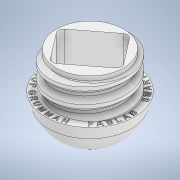
# Autodesk Inventor part: SmartEgg Shell
Saved by Autodesk Inventor 2020 (Build 240168000, 168)
## iProperties
Created: 2019-11-26
Part Number: SmartEgg Shell
Material: Generic
Document SubType Name: Modeling
Designer: Andrew
Density: 1 g/cm^3
Appearance: White
d0: 1.000 ul
d17: 1.000 ul
d18: 25.000 mm
d19: 50.000 mm
d20: 1.000 mm
d21: 17.000 mm
d22: 5.000 mm
d23: 2.000 mm
d24: 12.500 mm
d25: 0.250 mm
d26: 20.000 mm
d27: 3.000 mm
d28: 1.500 mm
d30: 1.000 mm
d32: 0.500 mm
d33: 0.500 mm
d35: 45.00 deg
d36: 0.250 mm
d37: 2.000 mm
d38: 2.000 mm
d41: 8.708 mm
d43: 3.000 ul
d44: 0.00 deg
d50: 8.708 mm
d52: 1.000 ul
d53: 0.00 deg
d61: 2.500 mm
d29: 70.533 mm
d39: 7.000 mm
Thread_Pitch: 4.354 mm
BATT_Width: 24.750 mm
PCB_Width: 22.950 mm
Author: Andrew
Autodesk Inventor part; units mm, degrees
ref_plane "YZ Plane" through (0, 0, 0) normal (1, 0, 0) x (0, 1, 0)
ref_plane "XZ Plane" through (0, 0, 0) normal (0, 1, 0) x (-1, 0, 0)
ref_plane "XY Plane" through (0, 0, 0) normal (0, 0, 1) x (1, 0, 0)
derived "SmartEgg Housing Main.ipt"
sketch "Sketch3" plane through (0, 0, 0) normal (0, 0, 1) x (1, 0, 0)
  line L0 (25.5, 9.7) -> (25.5, -9.55)
  line L1 (26.5, 11.95) -> (26.5, -11.8)
  line L2 (-26.5, -11.8) -> (-26.5, 11.95)
  line L3 (-7.3114, 6.9165) -> (-15.25, -6.8335)
  line L4 (-15.5, -6.7665) -> (-7.5614, 6.9835)
  line L5 (-26.5, 11.95) -> (-7.5614, 11.95)
  line L6 (-7.3114, 11.95) -> (26.5, 11.95)
  line L7 (-25.5, 9.7) -> (7.4386, 9.7)
  line L8 (7.6886, 9.7) -> (25.5, 9.7)
  line L9 (25.5, -9.55) -> (-0.25, -9.55)
  line L10 (-0.5, -9.55) -> (-25.5, -9.55)
  line L11 (26.5, -11.8) -> (-15.25, -11.8)
  line L12 (-15.5, -11.8) -> (-26.5, -11.8)
  line L13 (25.5, 0) -> (25.5, -1.8) construction
  line L14 (-25.5, -1.8) -> (-25.5, 0) construction
  line L15 (-25.5, -3.3) -> (-0.5, -3.3)
  line L16 (-0.5, -3.3) -> (-0.5, -4.3)
  line L17 (-0.5, -4.3) -> (-25.5, -4.3)
  line L18 (-25.5, -9.55) -> (-25.5, -4.3)
  line L19 (-25.5, -3.3) -> (-25.5, 9.7)
  line L20 (-7.4364, 11.95) -> (-7.4364, 6.95) construction
  line L21 (-7.4364, 6.95) -> (-15.375, -6.8) construction
  line L22 (-15.375, -6.8) -> (-15.375, -11.8) construction
  line L23 (-7.5614, 11.95) -> (-7.5614, 10.7)
  line L24 (-7.5614, 10.7) -> (7.4386, 10.7)
  line L25 (7.4386, 10.7) -> (7.4386, 9.7)
  line L26 (7.6886, 9.7) -> (7.6886, 10.95)
  line L27 (7.6886, 10.95) -> (-7.3114, 10.95)
  line L28 (-7.3114, 10.95) -> (-7.3114, 11.95)
  line L29 (-15.5, -11.8) -> (-15.5, -10.55)
  line L30 (-15.5, -10.55) -> (-0.5, -10.55)
  line L31 (-0.5, -10.55) -> (-0.5, -9.55)
  line L32 (-0.25, -9.55) -> (-0.25, -10.8)
  line L33 (-0.25, -10.8) -> (-15.25, -10.8)
  line L34 (-15.25, -10.8) -> (-15.25, -11.8)
  line L35 (-7.5614, 10.7) -> (-7.5614, 6.9835)
  line L36 (-7.3114, 6.9165) -> (-7.3114, 10.95)
  line L37 (-15.5, -10.55) -> (-15.5, -6.7665)
  line L38 (-15.25, -6.8335) -> (-15.25, -10.8)
  line L39 (7.4386, 9.7) -> (7.4386, 6.9835)
  line L40 (7.4386, 6.9835) -> (-0.5, -6.7665)
  line L41 (-0.5, -6.7665) -> (-0.5, -9.55)
  line L42 (-0.25, -9.55) -> (-0.25, -6.8335)
  line L43 (-0.25, -6.8335) -> (7.6886, 6.9165)
  line L44 (7.6886, 6.9165) -> (7.6886, 9.7)
  line L45 (-0.375, -11.8) -> (-0.375, -6.8) construction
  line L46 (-0.375, -6.8) -> (7.5636, 6.95) construction
  line L47 (7.5636, 6.95) -> (7.5636, 11.95) construction
  line L48 (11.5, -9.55) -> (16.5, -9.55)
  line L49 (16.5, -9.55) -> (14, -7.05)
  line L50 (14, -7.05) -> (11.5, -7.05)
  line L51 (11.5, -7.05) -> (11.5, -9.55)
  point P0 (0, 0)
derived "SmartEgg Housing Cap.ipt"
sketch "Housing Largest Area" plane through (0, -10.6204, -14.0095) normal (0, 0.7948428, -0.6068154) x (0, 0.6068154, 0.7948428)
  line L0 (30.7511, 26.5) -> (29.3995, 26.5)
  line L1 (17.6255, 26.5) -> (17.6255, -26.5)
  line L2 (17.6255, -26.5) -> (35.2511, -26.5)
  line L3 (35.2511, -26.5) -> (35.2511, 22)
  line L4 (10.4196, -26.5) -> (24.8315, -26.5) construction
  line L5 (24.8315, 26.5) -> (10.4196, 26.5) construction
  line L6 (12.0637, 20.5) -> (10.4158, 20.5) construction
  line L7 (10.4158, 20.5) -> (10.4158, 24.5) construction
  ellipse E0 centre (8.7678, 24.5) end of major axis (10.4158, 24.5) minor radius 1 (10.4158, 24.5) -> (8.7678, 25.5) ccw construction
  line L8 (8.7678, 25.5) -> (2.3515, 25.5) construction
  line L9 (2.3515, 25.5) -> (2.3515, 16.1435) construction
  line L10 (2.3515, -0.25) -> (1, -0.25) construction
  line L11 (1, -0.25) -> (1, -15.25) construction
  line L12 (1, -15.25) -> (0, -15.25) construction
  line L13 (0, -15.25) -> (0, 26.5) construction
  line L14 (17.0488, 25.5) -> (14.5356, 25.5) construction
  line L15 (14.5356, 25.5) -> (14.5356, 22.4142) construction
  ellipse E1 centre (12.8877, 22.4142) end of major axis (14.5356, 22.4142) minor radius 1 (14.053, 21.7071) -> (14.5356, 22.4142) ccw construction
  line L16 (14.053, 21.7071) -> (12.0637, 20.5) construction
  line L17 (35.2511, 26.5) -> (35.2511, -7.3114) construction
  line L18 (35.2511, -7.3114) -> (34.2511, -7.3114) construction
  line L19 (34.2511, -7.3114) -> (34.2511, 7.6886) construction
  line L20 (34.2511, 7.6886) -> (32.8995, 7.6886) construction
  line L21 (32.8995, 7.6886) -> (32.8995, 25.5) construction
  arc A0 (35.2511, 22) -> (30.7511, 26.5) centre (30.7511, 22) ccw
  arc A1 (32.8995, 22) -> (29.3995, 25.5) centre (29.3995, 22) ccw
  line L22 (32.8995, 22) -> (35.2511, 22)
  line L23 (29.3995, 25.5) -> (29.3995, 26.5)
  line L24 (29.3995, 26.5) -> (17.6255, 26.5)
  line L25 (2.3515, 16.1435) -> (4.5726, 14.7957)
  line L26 (4.5726, 14.7957) -> (4.5726, 11.5)
  line L27 (4.5726, 11.5) -> (2.3515, 11.5)
  line L28 (2.3515, 11.5) -> (2.3515, -0.25)
  line L29 (0, 26.5) -> (17.0488, 26.5)
  line L30 (17.0488, 26.5) -> (17.0488, 25.5)
  line L31 (32.8995, 25.5) -> (21.9926, 25.5)
  line L32 (21.9926, 25.5) -> (21.9926, 26.5)
  line L33 (21.9926, 26.5) -> (35.2511, 26.5)
  point P0 (17.58, 0)
  point P1 (17.6255, 0)
sketch "ESP32 Feather" plane through (0, 0, 0) normal (0, 0, 1) x (1, 0, 0)
  line L0 (-25.5, 0) -> (25.5, 0)
  line L1 (25.5, 0) -> (25.5, -1.8)
  line L2 (25.5, -1.8) -> (-25.5, -1.8)
  line L3 (-25.5, -1.8) -> (-25.5, 0)
  line L4 (0, 0) -> (-25.5, 0)
  line L5 (-25.5, 0) -> (-25.5, 0.75)
  line L6 (-25.5, 0.75) -> (0, 0.75)
  line L7 (0, 0.75) -> (0, 0)
  line L8 (-0.9, 0.75) -> (-18.55, 0.75)
  line L9 (-18.55, 0.75) -> (-18.55, 3.1)
  line L10 (-18.55, 3.1) -> (-0.9, 3.1)
  line L11 (-0.9, 3.1) -> (-0.9, 0.75)
  line L12 (10, 0) -> (18, 0)
  line L13 (18, 0) -> (18, 5.5)
  line L14 (18, 5.5) -> (10, 5.5)
  line L15 (10, 5.5) -> (10, 0)
  line L16 (25.6, 0) -> (19.95, 0)
  line L17 (19.95, 0) -> (19.95, 2.45)
  line L18 (19.95, 2.45) -> (25.6, 2.45)
  line L19 (25.6, 2.45) -> (25.6, 0)
  point P0 (0, 0)
  point P1 (0, 0)
  point P2 (-18.55, 0.75)
  point P3 (18, 0)
  point P4 (19.95, 0)
sketch "Shell Sketch" plane through (0, -10.6204, -14.0095) normal (0, 0.7948428, -0.6068154) x (0, 0.6068154, 0.7948428)
  arc A0 (41.0761, -18.875) -> (29.7061, 33.6321) centre (-5.8251, -1.5465) ccw
  arc A1 (17.6255, -35.2107) -> (30.1255, -31.8614) centre (17.6255, -10.2107) ccw construction
  line L0 (17.6255, -35.2107) -> (17.6255, -31.8614) construction
  line L1 (17.6255, 9) -> (36.7511, 9)
  line L2 (17.6255, 26.5) -> (17.6255, -26.5) construction
  line L3 (35.2511, -26.5) -> (35.9855, -27.1787) construction
  arc A2 (29.7061, 33.6321) -> (17.6255, 38.6714) centre (17.6255, 21.6714) ccw
  line L4 (17.6255, 38.6714) -> (17.6255, 35.8135)
  line L5 (17.6255, 35.8135) -> (22.6255, 35.8135)
  arc A3 (28.2849, 32.225) -> (22.6255, 35.8135) centre (17.6255, 21.6714) ccw
  arc A4 (37.3586, 19.41) -> (28.2849, 32.225) centre (-5.8251, -1.5465) ccw
  arc A5 (35.2511, 22) -> (30.7511, 26.5) centre (30.7511, 22) ccw construction
  line L6 (36.7511, 9) -> (36.7511, -11.8614)
  line L7 (36.7511, -11.8614) -> (43.0994, -11.8614)
  line L8 (39.7511, 9) -> (39.7511, -11.6114)
  line L9 (39.7511, -11.6114) -> (43.1514, -11.6114)
  line L10 (17.6255, -31.8614) -> (30.1255, -31.8614)
  arc A6 (30.1255, -31.8614) -> (41.0761, -18.875) centre (17.6255, -10.2107) ccw
  line L11 (17.6255, -31.8614) -> (17.6255, 9)
  line L12 (35.2511, -26.5) -> (35.2511, 22) construction
  line L13 (20.9175, 10) -> (17.58, 10) construction
  arc A7 (39.7511, 9) -> (37.3586, 19.41) centre (15.9074, 9) ccw
  point P0 (17.58, 0)
  point P1 (39.7511, 13.5139)
  dimension "d18" = 25
  dimension "d19" = 50
  dimension "d20" = 1
  dimension "d21" = 17
  dimension "d22" = 5
  dimension "d23" = 2
  dimension "d24" = 12.5
  dimension "d25" = 0.25
  dimension "d26" = 20
  dimension "d27" = 3
  dimension "d28" = 1.5
  dimension "d29" = 70.5327
  dimension "d30" = 1
  constraints: 22 end point, 19 point on circle, 7 centre point, 7 line through centre, 6 perpendicular, 6 tangent, 4 collinear, 4 vertical, 2 concentric, 2 point on line, 1 coincident, 1 horizontal
  measures "d18" radius of A1
  measures "d19" radius of A0
  measures "d20" distance of L3.start L3.end
  measures "d21" radius of A2
  measures "d22" distance of L4.end L5.end
  measures "d23" radial gap between concentric circles of A0 A4
  measures "d24" distance of L0.end L10.end
  measures "d25" distance between parallel lines of L7 L9
  measures "d26" distance between parallel lines of L10 L7
  measures "d27" distance between parallel lines of L8 L6
  measures "d28" distance between parallel lines of L12 L6
  measures "d29" distance from line of L10 L4.start
  measures "d30" distance between parallel lines of L1 L13
sketch "Thread Sketch" plane through (0, -10.6204, -14.0095) normal (0, 0.7948428, -0.6068154) x (0, 0.6068154, 0.7948428)
  line L0 (36.7511, 9) -> (36.7511, -11.8614) construction
  line L1 (39.7511, 9) -> (39.7511, -11.6114) construction
  line L2 (36.7511, 9) -> (39.2511, 6.5)
  line L3 (39.2511, 6.5) -> (39.2511, 4.5)
  line L4 (39.2511, 4.5) -> (36.7511, 2)
  line L5 (36.7511, 2) -> (36.7511, 9)
  line L6 (39.7511, 4.6464) -> (37.2511, 2.1464)
  line L7 (37.2511, 2.1464) -> (37.2511, 0.1464)
  line L8 (37.2511, 0.1464) -> (39.7511, -2.3536)
  line L9 (39.7511, -2.3536) -> (39.7511, 4.6464)
  line L10 (39.2511, 5.5) -> (36.7511, 5.5) construction
  line L11 (37.2511, 1.1464) -> (39.7511, 1.1464) construction
  point P0 (17.58, 0)
  dimension "d32" = 0.5
  dimension "d33" = 0.5
  dimension "d35" = 45
  dimension "d36" = 0.25
  dimension "d37" = 2
  dimension "d38" = 2
  dimension "d39" = 7
  dimension "Thread_Pitch" = 4.354
  constraints: 20 end point, 4 midpoint, 3 parallel, 2 horizontal, 2 point on line, 2 other
  measures "d32" distance between parallel lines of L1 L3
  measures "d33" distance between parallel lines of L0 L7
  measures "d35" angle of L0 L4
  measures "d36" distance between parallel lines of L6 L4
  measures "d37" distance of L2.end L3.end
  measures "d38" distance of L6.end L7.end
  measures "d39" distance of L4.end L0.start
revolve "Revolution1" add sketch "Shell Sketch" angle 360 about axis through (-31.8614, 0.075, 0) along (1, 0, 0) contours A6 L10 L11 L1 L6 L7 A0
coil "Coil1" sketch "Thread Sketch" operation add axis through (-31.8614, 0.075, 0) along (-1, 0, 0) pitch 8.708 turns 3 hand right separate body contours L2 L3 L4 L5
coil "Coil2" sketch "Thread Sketch" operation add axis through (-31.8614, 0.075, 0) along (1, 0, 0) pitch 8.708 turns 1 hand right bodies 2 contours L2 L3 L4 L5
sketch "Thread Mask" plane through (0, -10.6204, -14.0095) normal (0, 0.7948428, -0.6068154) x (0, 0.6068154, 0.7948428)
  line L0 (39.7511, 6.5) -> (36.7511, 6.5)
  line L1 (36.7511, 6.5) -> (36.7511, -11.8614)
  line L2 (36.7511, -11.8614) -> (39.7511, -11.8614)
  line L3 (39.7511, -11.8614) -> (39.7511, 6.5)
  line L4 (36.7511, 9) -> (36.7511, -11.8614) construction
  line L5 (39.7511, 9) -> (39.7511, -11.6114) construction
  point P0 (17.58, 0)
  dimension "d61" = 2.5
  constraints: 8 end point, 2 parallel, 1 collinear, 1 horizontal, 1 perpendicular
  measures "d61" distance from line of L4.start L0
revolve "Revolution4" cut sketch "Thread Mask" angle 360 about axis through (-31.8614, 0.075, 0) along (1, 0, 0) keep common part bodies 2
combine bodies "Combine1" operation type add bodies to combine 1 2
sketch "Sketch10" plane through (9, 0.075, 0) normal (1, 0, 0) x (0, 0, -1)
  line L0 (-11.875, -12.125) -> (11.875, -12.125)
  line L1 (14.875, -9.125) -> (14.875, 9.125)
  line L2 (11.875, 12.125) -> (-11.875, 12.125)
  line L3 (-14.875, 9.125) -> (-14.875, -9.125)
  line L4 (-14.875, 0) -> (14.875, 0) construction
  arc A0 (-11.875, 12.125) -> (-14.875, 9.125) centre (-11.875, 9.125) ccw
  arc A1 (14.875, 9.125) -> (11.875, 12.125) centre (11.875, 9.125) ccw
  arc A2 (11.875, -12.125) -> (14.875, -9.125) centre (11.875, -9.125) ccw
  arc A3 (-14.875, -9.125) -> (-11.875, -12.125) centre (-11.875, -9.125) ccw
  point P0 (0, -0.075)
  point P1 (14.875, 12.125)
  point P2 (-14.875, 12.125)
  point P3 (0, -11.875)
  point P4 (0, -11.875)
  point P5 (0, -11.875)
  point P6 (0, 11.875)
  point P7 (0, 11.875)
  point P8 (0, 11.875)
  point P9 (0, 0)
  point P10 (0, 0)
  point P11 (0, 0)
  point P12 (0, 0)
  dimension "d64" = 0.25
  dimension "d65" = 29.75
  dimension "d66" = 3
  constraints: 10 end point, 8 point on circle, 8 tangent, 4 centre point, 4 point on line, 3 equal radius, 3 midpoint, 2 parallel, 1 coincident, 1 horizontal, 1 perpendicular
  measures "d64" distance from line of L0 point (0, -11.875)
  measures "d65" distance of point (14.875, 12.125) point (-14.875, 12.125)
  measures "d66" radius of A0
sketch "Sketch11" plane through (0, 0, 0) normal (0, 0, 1) x (1, 0, 0)
  line L0 (9, 19.2005) -> (9, -19.0505) projected
  line L1 (9, 0.075) -> (-26.5, 0.075)
  line L2 (-26.5, -11.8) -> (-26.5, 11.95) construction
  point P0 (0, 0)
  dimension "d67" = 35.5
  constraints: 2 end point, 2 midpoint, 1 horizontal
  measures "d67" distance of L1.start L1.end
extrude "Extrusion1" cut sketch "Sketch10" against normal blind 35.5 bodies 1
sketch "Vent Lookup" plane through (0, -10.6204, -14.0095) normal (0, 0.7948428, -0.6068154) x (0, 0.6068154, 0.7948428)
  arc A0 (41.0761, -18.875) -> (29.7061, 33.6321) centre (-5.8251, -1.5465) ccw projected
  line L0 (40.8046, 16.5) -> (17.6255, 7.5293)
  line L1 (17.6255, 26.5) -> (17.6255, -26.5) construction
  line L2 (20.9175, 10) -> (17.58, 10) construction
  point P0 (17.58, 0)
  dimension "d71" = 6.5
  constraints: 2 end point, 1 line through centre, 1 point on circle, 1 point on line
  measures "d71" distance from line of L2 L0.start
ref_plane "Vent Plane" through (16.5, 14.1404, 18.4237) normal (-0.3609294, -0.5659119, -0.7412649) x (0.8431188, -0.5377274, 0)
sketch "Sketch13" plane through (-11.8614, 0.075, 0) normal (1, 0, 0) x (0, 0, -1)
  circle A0 centre (0, -0.075) radius 24.75 construction
  line L0 (7.0609, -23.8279) -> (6.0494, -20.9526)
  line L1 (6.0494, -20.9526) -> (6.6126, -20.7545)
  line L2 (6.6126, -20.7545) -> (8.4723, -22.2675)
  line L3 (8.4723, -22.2675) -> (7.7938, -20.3389)
  line L4 (7.7938, -20.3389) -> (8.3307, -20.15)
  line L5 (8.3307, -20.15) -> (9.3423, -23.0253)
  line L6 (9.3423, -23.0253) -> (8.7615, -23.2296)
  line L7 (8.7615, -23.2296) -> (6.934, -21.7521)
  line L8 (6.934, -21.7521) -> (7.5978, -23.639)
  line L9 (7.5978, -23.639) -> (7.0609, -23.8279)
  spline S0 degree 2 poles (10.1675, -21.0296) (9.9387, -20.6252) (9.9044, -20.2816) knots 0 0 0 1 1 1
  spline S1 degree 2 poles (9.9044, -20.2816) (9.881, -20.0279) (10.0113, -19.5271) (10.1539, -19.345) knots 0 0 0 1 2 2 2
  spline S2 degree 2 poles (10.1539, -19.345) (10.3411, -19.1002) (10.6666, -18.916) knots 0 0 0 1 1 1
  spline S3 degree 2 poles (10.6666, -18.916) (11.2529, -18.5843) (12.3685, -18.914) (12.7346, -19.561) knots 0 0 0 1 2 2 2
  spline S4 degree 2 poles (12.7346, -19.561) (13.0972, -20.202) (12.8084, -21.3237) (12.2241, -21.6543) knots 0 0 0 1 2 2 2
  spline S5 degree 2 poles (12.2241, -21.6543) (11.6337, -21.9884) (10.5256, -21.6624) (10.1675, -21.0296) knots 0 0 0 1 2 2 2
  spline S6 degree 2 poles (10.7092, -20.699) (10.9644, -21.1499) (11.644, -21.3793) (11.9655, -21.1974) knots 0 0 0 1 2 2 2
  spline S7 degree 2 poles (11.9655, -21.1974) (12.287, -21.0155) (12.4366, -20.3222) (12.1757, -19.8612) knots 0 0 0 1 2 2 2
  spline S8 degree 2 poles (12.1757, -19.8612) (11.9171, -19.4043) (11.2628, -19.1819) (10.9312, -19.3696) knots 0 0 0 1 2 2 2
  spline S9 degree 2 poles (10.9312, -19.3696) (10.5996, -19.5572) (10.4506, -20.2421) (10.7092, -20.699) knots 0 0 0 1 2 2 2
  line L10 (14.8398, -19.9206) -> (12.8959, -17.5729)
  line L11 (12.8959, -17.5729) -> (13.8943, -16.7462)
  spline S10 degree 2 poles (13.8943, -16.7462) (14.2719, -16.4336) (14.7171, -16.2791) (15.1896, -16.4308) (15.3629, -16.6402) knots 0 0 0 1 2 3 3 3
  spline S11 degree 2 poles (15.3629, -16.6402) (15.5807, -16.9032) (15.5571, -17.5049) (15.2846, -17.8059) knots 0 0 0 1 2 2 2
  spline S12 degree 2 poles (15.2846, -17.8059) (15.5125, -17.768) (15.8908, -17.8168) (16.2874, -17.9498) knots 0 0 0 1 2 2 2
  line L12 (16.2874, -17.9498) -> (16.953, -18.1708)
  line L13 (16.953, -18.1708) -> (16.3858, -18.6405)
  line L14 (16.3858, -18.6405) -> (15.6203, -18.4117)
  spline S13 degree 2 poles (15.6203, -18.4117) (15.2093, -18.2905) (14.9565, -18.2585) (14.7633, -18.3311) (14.5986, -18.4674) knots 0 0 0 1 2 3 3 3
  line L15 (14.5986, -18.4674) -> (14.502, -18.5474)
  line L16 (14.502, -18.5474) -> (15.314, -19.528)
  line L17 (15.314, -19.528) -> (14.8398, -19.9206)
  line L18 (14.1924, -18.1734) -> (14.5431, -17.883)
  spline S14 degree 2 poles (14.5431, -17.883) (14.8849, -17.6) (15.0074, -17.402) (14.987, -17.1806) (14.8996, -17.0751) knots 0 0 0 1 2 3 3 3
  spline S15 degree 2 poles (14.8996, -17.0751) (14.8018, -16.957) (14.5533, -16.9154) (14.4225, -16.9906) knots 0 0 0 1 2 2 2
  spline S16 degree 2 poles (14.4225, -16.9906) (14.3575, -17.0323) (14.0694, -17.2709) knots 0 0 0 1 1 1
  line L19 (14.0694, -17.2709) -> (13.699, -17.5776)
  line L20 (13.699, -17.5776) -> (14.1924, -18.1734)
  line L21 (18.4583, -16.5658) -> (16.5493, -14.902)
  line L22 (16.5493, -14.902) -> (15.9555, -15.5833)
  line L23 (15.9555, -15.5833) -> (15.5667, -15.2445)
  line L24 (15.5667, -15.2445) -> (17.1572, -13.4195)
  line L25 (17.1572, -13.4195) -> (17.546, -13.7584)
  line L26 (17.546, -13.7584) -> (16.9538, -14.4379)
  line L27 (16.9538, -14.4379) -> (18.8628, -16.1017)
  line L28 (18.8628, -16.1017) -> (18.4583, -16.5658)
  line L29 (20.3954, -14.1496) -> (17.8041, -12.5447)
  line L30 (17.8041, -12.5447) -> (18.1283, -12.0213)
  line L31 (18.1283, -12.0213) -> (19.1474, -12.6525)
  line L32 (19.1474, -12.6525) -> (19.7823, -11.6275)
  line L33 (19.7823, -11.6275) -> (18.7632, -10.9963)
  line L34 (18.7632, -10.9963) -> (19.0873, -10.4729)
  line L35 (19.0873, -10.4729) -> (21.6786, -12.0778)
  line L36 (21.6786, -12.0778) -> (21.3544, -12.6012)
  line L37 (21.3544, -12.6012) -> (20.2207, -11.899)
  line L38 (20.2207, -11.899) -> (19.5859, -12.9241)
  line L39 (19.5859, -12.9241) -> (20.7196, -13.6262)
  line L40 (20.7196, -13.6262) -> (20.3954, -14.1496)
  line L41 (22.5022, -10.4537) -> (19.6746, -9.3157)
  line L42 (19.6746, -9.3157) -> (20.1586, -8.1131)
  spline S17 degree 2 poles (20.1586, -8.1131) (20.3416, -7.6584) (20.6595, -7.3105) (21.1471, -7.2188) (21.3993, -7.3203) knots 0 0 0 1 2 3 3 3
  spline S18 degree 2 poles (21.3993, -7.3203) (21.7161, -7.4478) (21.982, -7.988) (21.8858, -8.3826) knots 0 0 0 1 2 2 2
  spline S19 degree 2 poles (21.8858, -8.3826) (22.0682, -8.2406) (22.4239, -8.1033) (22.8361, -8.0313) knots 0 0 0 1 2 2 2
  line L43 (22.8361, -8.0313) -> (23.5266, -7.9085)
  line L44 (23.5266, -7.9085) -> (23.2516, -8.5917)
  line L45 (23.2516, -8.5917) -> (22.4696, -8.7552)
  spline S20 degree 2 poles (22.4696, -8.7552) (22.0505, -8.8445) (21.813, -8.9368) (21.6777, -9.0926) (21.5979, -9.2909) knots 0 0 0 1 2 3 3 3
  line L46 (21.5979, -9.2909) -> (21.551, -9.4073)
  line L47 (21.551, -9.4073) -> (22.7321, -9.8826)
  line L48 (22.7321, -9.8826) -> (22.5022, -10.4537)
  line L49 (21.1006, -9.226) -> (21.2706, -8.8036)
  spline S21 degree 2 poles (21.2706, -8.8036) (21.4363, -8.392) (21.4497, -8.1595) (21.3263, -7.9746) (21.1991, -7.9234) knots 0 0 0 1 2 3 3 3
  spline S22 degree 2 poles (21.1991, -7.9234) (21.0569, -7.8661) (20.8186, -7.948) (20.7394, -8.0764) knots 0 0 0 1 2 2 2
  spline S23 degree 2 poles (20.7394, -8.0764) (20.7021, -8.1441) (20.5625, -8.491) knots 0 0 0 1 1 1
  line L50 (20.5625, -8.491) -> (20.3829, -8.9372)
  line L51 (20.3829, -8.9372) -> (21.1006, -9.226)
  spline S24 degree 2 poles (22.4524, -6.2686) (21.9976, -6.1736) (21.7169, -5.9725) knots 0 0 0 1 1 1
  spline S25 degree 2 poles (21.7169, -5.9725) (21.5108, -5.8227) (21.2206, -5.3942) (21.1779, -5.1669) knots 0 0 0 1 2 2 2
  spline S26 degree 2 poles (21.1779, -5.1669) (21.1177, -4.8648) (21.1942, -4.4987) knots 0 0 0 1 1 1
  spline S27 degree 2 poles (21.1942, -4.4987) (21.332, -3.8392) (22.316, -3.2189) (23.0437, -3.3709) knots 0 0 0 1 2 2 2
  spline S28 degree 2 poles (23.0437, -3.3709) (23.7645, -3.5215) (24.4165, -4.4789) (24.2792, -5.1361) knots 0 0 0 1 2 2 2
  spline S29 degree 2 poles (24.2792, -5.1361) (24.1405, -5.8002) (23.1642, -6.4174) (22.4524, -6.2686) knots 0 0 0 1 2 2 2
  spline S30 degree 2 poles (22.5617, -5.6435) (23.0688, -5.7495) (23.6897, -5.3903) (23.7653, -5.0288) knots 0 0 0 1 2 2 2
  spline S31 degree 2 poles (23.7653, -5.0288) (23.8408, -4.6672) (23.4188, -4.0972) (22.9003, -3.9889) knots 0 0 0 1 2 2 2
  spline S32 degree 2 poles (22.9003, -3.9889) (22.3864, -3.8815) (21.7874, -4.2263) (21.7095, -4.5992) knots 0 0 0 1 2 2 2
  spline S33 degree 2 poles (21.7095, -4.5992) (21.6316, -4.9722) (22.0478, -5.5362) (22.5617, -5.6435) knots 0 0 0 1 2 2 2
  line L52 (24.6979, -2.0263) -> (21.6517, -1.9225)
  line L53 (21.6517, -1.9225) -> (21.6853, -0.9357)
  spline S34 degree 2 poles (21.6853, -0.9357) (21.7044, -0.3738) (21.7566, -0.2059) knots 0 0 0 1 1 1
  spline S35 degree 2 poles (21.7566, -0.2059) (21.8329, 0.0542) (22.3046, 0.3914) (22.6692, 0.379) knots 0 0 0 1 2 2 2
  spline S36 degree 2 poles (22.6692, 0.379) (22.9478, 0.3695) (23.3239, 0.1521) (23.5315, -0.1687) (23.5608, -0.3325) knots 0 0 0 1 2 3 3 3
  spline S37 degree 2 poles (23.5608, -0.3325) (23.5975, -0.5522) (23.5832, -0.9701) knots 0 0 0 1 1 1
  line L54 (23.5832, -0.9701) -> (23.5695, -1.3718)
  line L55 (23.5695, -1.3718) -> (24.7188, -1.411)
  line L56 (24.7188, -1.411) -> (24.6979, -2.0263)
  line L57 (22.1881, -1.3248) -> (23.0541, -1.3543)
  line L58 (23.0541, -1.3543) -> (23.0656, -1.0176)
  spline S38 degree 2 poles (23.0656, -1.0176) (23.078, -0.6531) (22.9911, -0.406) (22.7915, -0.2598) (22.6569, -0.2552) knots 0 0 0 1 2 3 3 3
  spline S39 degree 2 poles (22.6569, -0.2552) (22.4897, -0.2495) (22.2671, -0.4372) (22.2341, -0.5871) knots 0 0 0 1 2 2 2
  spline S40 degree 2 poles (22.2341, -0.5871) (22.2095, -0.6955) (22.1982, -1.0276) knots 0 0 0 1 1 1
  line L59 (22.1982, -1.0276) -> (22.1881, -1.3248)
  line L60 (23.2132, 4.358) -> (22.7063, 4.2628)
  line L61 (22.7063, 4.2628) -> (22.4614, 5.5665)
  line L62 (22.4614, 5.5665) -> (23.6533, 5.7904)
  spline S41 degree 2 poles (23.6533, 5.7904) (23.8738, 5.6356) (24.2879, 4.9664) (24.3574, 4.5965) knots 0 0 0 1 2 2 2
  spline S42 degree 2 poles (24.3574, 4.5965) (24.4457, 4.1262) (24.1819, 3.3533) (23.515, 2.864) (23.0858, 2.7834) knots 0 0 0 1 2 3 3 3
  spline S43 degree 2 poles (23.0858, 2.7834) (22.6177, 2.6955) (21.8156, 2.9514) (21.5508, 3.2917) knots 0 0 0 1 2 2 2
  spline S44 degree 2 poles (21.5508, 3.2917) (21.3479, 3.5538) (21.2673, 3.9831) knots 0 0 0 1 1 1
  spline S45 degree 2 poles (21.2673, 3.9831) (21.1626, 4.5402) (21.5128, 5.256) (21.9093, 5.4226) knots 0 0 0 1 2 2 2
  line L63 (21.9093, 5.4226) -> (22.134, 4.8432)
  spline S46 degree 2 poles (22.134, 4.8432) (21.9245, 4.7376) (21.7344, 4.3403) (21.7833, 4.08) knots 0 0 0 1 2 2 2
  spline S47 degree 2 poles (21.7833, 4.08) (21.8579, 3.6827) (22.4481, 3.309) (22.9436, 3.402) knots 0 0 0 1 2 2 2
  spline S48 degree 2 poles (22.9436, 3.402) (23.4756, 3.5019) (23.9207, 4.0772) (23.8486, 4.4608) knots 0 0 0 1 2 2 2
  spline S49 degree 2 poles (23.8486, 4.4608) (23.813, 4.6503) (23.593, 5.0037) (23.4623, 5.121) knots 0 0 0 1 2 2 2
  line L64 (23.4623, 5.121) -> (23.0832, 5.0498)
  line L65 (23.0832, 5.0498) -> (23.2132, 4.358)
  line L66 (23.5781, 7.5501) -> (20.7279, 6.4698)
  line L67 (20.7279, 6.4698) -> (20.2685, 7.682)
  spline S50 degree 2 poles (20.2685, 7.682) (20.0947, 8.1403) (20.0925, 8.6116) (20.3889, 9.0096) (20.643, 9.1059) knots 0 0 0 1 2 3 3 3
  spline S51 degree 2 poles (20.643, 9.1059) (20.9624, 9.227) (21.5241, 9.0101) (21.7208, 8.6548) knots 0 0 0 1 2 2 2
  spline S52 degree 2 poles (21.7208, 8.6548) (21.7586, 8.8828) (21.9271, 9.2249) (22.1812, 9.5573) knots 0 0 0 1 2 2 2
  line L68 (22.1812, 9.5573) -> (22.6056, 10.1157)
  line L69 (22.6056, 10.1157) -> (22.8666, 9.427)
  line L70 (22.8666, 9.427) -> (22.4026, 8.7766)
  spline S53 degree 2 poles (22.4026, 8.7766) (22.1551, 8.4269) (22.043, 8.1981) (22.0492, 7.9917) (22.1249, 7.7919) knots 0 0 0 1 2 3 3 3
  line L71 (22.1249, 7.7919) -> (22.1694, 7.6746)
  line L72 (22.1694, 7.6746) -> (23.3599, 8.1258)
  line L73 (23.3599, 8.1258) -> (23.5781, 7.5501)
  line L74 (21.7154, 7.5025) -> (21.554, 7.9282)
  spline S54 degree 2 poles (21.554, 7.9282) (21.3967, 8.3432) (21.249, 8.5232) (21.0329, 8.5755) (20.9047, 8.5269) knots 0 0 0 1 2 3 3 3
  spline S55 degree 2 poles (20.9047, 8.5269) (20.7614, 8.4725) (20.6417, 8.2508) (20.6705, 8.1027) knots 0 0 0 1 2 2 2
  spline S56 degree 2 poles (20.6705, 8.1027) (20.689, 8.0277) (20.8215, 7.678) knots 0 0 0 1 1 1
  line L75 (20.8215, 7.678) -> (20.992, 7.2283)
  line L76 (20.992, 7.2283) -> (21.7154, 7.5025)
  line L77 (19.3054, 9.9147) -> (18.992, 10.4446)
  line L78 (18.992, 10.4446) -> (20.4136, 11.2856)
  spline S57 degree 2 poles (20.4136, 11.2856) (20.7515, 11.4855) (20.8397, 11.5646) knots 0 0 0 1 1 1
  spline S58 degree 2 poles (20.8397, 11.5646) (20.9795, 11.6932) (21.0241, 12.0651) (20.8928, 12.287) knots 0 0 0 1 2 2 2
  spline S59 degree 2 poles (20.8928, 12.287) (20.7603, 12.511) (20.4403, 12.6321) (20.1452, 12.5196) (19.8333, 12.335) knots 0 0 0 1 2 3 3 3
  line L79 (19.8333, 12.335) -> (18.3816, 11.4763)
  line L80 (18.3816, 11.4763) -> (18.0682, 12.0062)
  line L81 (18.0682, 12.0062) -> (19.4458, 12.8212)
  spline S60 degree 2 poles (19.4458, 12.8212) (19.9177, 13.1003) (20.3585, 13.245) (20.7624, 13.1735) (21.1519, 12.8802) (21.3352, 12.5703) knots 0 0 0 1 2 3 4 4 4
  spline S61 degree 2 poles (21.3352, 12.5703) (21.5576, 12.1944) (21.6131, 11.7036) (21.4708, 11.3144) (21.3381, 11.1874) knots 0 0 0 1 2 3 3 3
  spline S62 degree 2 poles (21.3381, 11.1874) (21.145, 11.0029) (20.7051, 10.7427) knots 0 0 0 1 1 1
  line L82 (20.7051, 10.7427) -> (19.3054, 9.9147)
  line L83 (19.6434, 15.053) -> (17.343, 13.0534)
  line L84 (17.343, 13.0534) -> (16.738, 13.7495)
  line L85 (16.738, 13.7495) -> (17.946, 15.5291)
  line L86 (17.946, 15.5291) -> (16.0216, 14.5736)
  line L87 (16.0216, 14.5736) -> (15.4151, 15.2714)
  line L88 (15.4151, 15.2714) -> (17.7155, 17.271)
  line L89 (17.7155, 17.271) -> (18.0889, 16.8414)
  line L90 (18.0889, 16.8414) -> (16.2776, 15.2671)
  line L91 (16.2776, 15.2671) -> (18.4851, 16.3856)
  line L92 (18.4851, 16.3856) -> (18.8753, 15.9367)
  line L93 (18.8753, 15.9367) -> (17.4573, 13.91)
  line L94 (17.4573, 13.91) -> (19.27, 15.4826)
  line L95 (19.27, 15.4826) -> (19.6434, 15.053)
  line L96 (16.417, 18.5047) -> (14.5377, 16.105)
  line L97 (14.5377, 16.105) -> (13.8115, 16.6737)
  line L98 (13.8115, 16.6737) -> (14.6601, 18.6501)
  line L99 (14.6601, 18.6501) -> (12.9519, 17.3469)
  line L100 (12.9519, 17.3469) -> (12.2239, 17.917)
  line L101 (12.2239, 17.917) -> (14.1032, 20.3167)
  line L102 (14.1032, 20.3167) -> (14.5514, 19.9657)
  line L103 (14.5514, 19.9657) -> (13.0717, 18.0763)
  line L104 (13.0717, 18.0763) -> (15.0269, 19.5933)
  line L105 (15.0269, 19.5933) -> (15.4951, 19.2266)
  line L106 (15.4951, 19.2266) -> (14.4874, 16.9677)
  line L107 (14.4874, 16.9677) -> (15.9689, 18.8556)
  line L108 (15.9689, 18.8556) -> (16.417, 18.5047)
  line L109 (10.1495, 22.5493) -> (10.742, 22.2386)
  line L110 (10.742, 22.2386) -> (10.655, 21.5025)
  line L111 (10.655, 21.5025) -> (11.7331, 20.9371)
  line L112 (11.7331, 20.9371) -> (12.2789, 21.4326)
  line L113 (12.2789, 21.4326) -> (12.857, 21.1294)
  line L114 (12.857, 21.1294) -> (10.3921, 18.9803)
  line L115 (10.3921, 18.9803) -> (9.8119, 19.2846)
  line L116 (9.8119, 19.2846) -> (10.1495, 22.5493)
  line L117 (10.5903, 20.954) -> (10.4383, 19.7588)
  line L118 (10.4383, 19.7588) -> (11.3289, 20.5666)
  line L119 (11.3289, 20.5666) -> (10.5903, 20.954)
  line L120 (8.7399, 23.1127) -> (7.8069, 20.211)
  line L121 (7.8069, 20.211) -> (7.2385, 20.3938)
  line L122 (7.2385, 20.3938) -> (6.6722, 22.7234)
  line L123 (6.6722, 22.7234) -> (6.0464, 20.7771)
  line L124 (6.0464, 20.7771) -> (5.5045, 20.9514)
  line L125 (5.5045, 20.9514) -> (6.4376, 23.853)
  line L126 (6.4376, 23.853) -> (7.0237, 23.6646)
  line L127 (7.0237, 23.6646) -> (7.5857, 21.3827)
  line L128 (7.5857, 21.3827) -> (8.1981, 23.2869)
  line L129 (8.1981, 23.2869) -> (8.7399, 23.1127)
  line L130 (-2.4203, 24.5762) -> (-2.0015, 21.5572)
  line L131 (-2.0015, 21.5572) -> (-4.0749, 21.2696)
  line L132 (-4.0749, 21.2696) -> (-4.1457, 21.7804)
  line L133 (-4.1457, 21.7804) -> (-2.6822, 21.9834)
  line L134 (-2.6822, 21.9834) -> (-2.7811, 22.6968)
  line L135 (-2.7811, 22.6968) -> (-4.0445, 22.5215)
  line L136 (-4.0445, 22.5215) -> (-4.1153, 23.0324)
  line L137 (-4.1153, 23.0324) -> (-2.852, 23.2076)
  line L138 (-2.852, 23.2076) -> (-3.0301, 24.4917)
  line L139 (-3.0301, 24.4917) -> (-2.4203, 24.5762)
  line L140 (-8.7698, 23.119) -> (-8.1306, 23.3169)
  line L141 (-8.1306, 23.3169) -> (-7.6729, 22.7338)
  line L142 (-7.6729, 22.7338) -> (-6.51, 23.0938)
  line L143 (-6.51, 23.0938) -> (-6.4728, 23.83)
  line L144 (-6.4728, 23.83) -> (-5.8492, 24.023)
  line L145 (-5.8492, 24.023) -> (-6.0797, 20.761)
  line L146 (-6.0797, 20.761) -> (-6.7056, 20.5673)
  line L147 (-6.7056, 20.5673) -> (-8.7698, 23.119)
  line L148 (-7.3318, 22.2995) -> (-6.5962, 21.3453)
  line L149 (-6.5962, 21.3453) -> (-6.535, 22.5461)
  line L150 (-6.535, 22.5461) -> (-7.3318, 22.2995)
  line L151 (-8.776, 19.8113) -> (-9.8623, 19.2566)
  spline S63 degree 2 poles (-9.8623, 19.2566) (-10.185, 19.0918) (-10.5291, 18.984) (-10.8661, 19.0259) (-11.1784, 19.2237) (-11.2682, 19.3996) knots 0 0 0 1 2 3 4 4 4
  spline S64 degree 2 poles (-11.2682, 19.3996) (-11.3654, 19.59) (-11.3222, 20.0111) (-11.1875, 20.1816) knots 0 0 0 1 2 2 2
  spline S65 degree 2 poles (-11.1875, 20.1816) (-11.4728, 20.1273) (-11.9151, 20.3397) (-12.0355, 20.5755) knots 0 0 0 1 2 2 2
  spline S66 degree 2 poles (-12.0355, 20.5755) (-12.1306, 20.7618) (-12.1374, 21.1991) (-11.9441, 21.5613) (-11.7395, 21.697) knots 0 0 0 1 2 3 3 3
  spline S67 degree 2 poles (-11.7395, 21.697) (-11.6082, 21.7823) (-11.0869, 22.0537) knots 0 0 0 1 1 1
  line L152 (-11.0869, 22.0537) -> (-10.162, 22.5259)
  line L153 (-10.162, 22.5259) -> (-8.776, 19.8113)
  line L154 (-10.105, 21.0604) -> (-10.4758, 21.7866)
  line L155 (-10.4758, 21.7866) -> (-10.9848, 21.5267)
  spline S68 degree 2 poles (-10.9848, 21.5267) (-11.2827, 21.3746) (-11.3529, 21.3179) knots 0 0 0 1 1 1
  spline S69 degree 2 poles (-11.3529, 21.3179) (-11.4634, 21.2328) (-11.5309, 20.9819) (-11.4569, 20.837) knots 0 0 0 1 2 2 2
  spline S70 degree 2 poles (-11.4569, 20.837) (-11.3946, 20.715) (-11.19, 20.6055) (-10.9243, 20.642) (-10.5498, 20.8332) knots 0 0 0 1 2 3 3 3
  line L156 (-10.5498, 20.8332) -> (-10.105, 21.0604)
  line L157 (-9.5546, 19.9824) -> (-9.8747, 20.6093)
  line L158 (-9.8747, 20.6093) -> (-10.2347, 20.4255)
  spline S71 degree 2 poles (-10.2347, 20.4255) (-10.5554, 20.2617) (-10.6298, 20.2133) knots 0 0 0 1 1 1
  spline S72 degree 2 poles (-10.6298, 20.2133) (-10.761, 20.1229) (-10.8411, 19.8812) (-10.7734, 19.7487) knots 0 0 0 1 2 2 2
  spline S73 degree 2 poles (-10.7734, 19.7487) (-10.709, 19.6225) (-10.4911, 19.5381) (-10.343, 19.5903) knots 0 0 0 1 2 2 2
  spline S74 degree 2 poles (-10.343, 19.5903) (-10.2581, 19.6232) (-9.8691, 19.8218) knots 0 0 0 1 1 1
  line L159 (-9.8691, 19.8218) -> (-9.5546, 19.9824)
  line L160 (-13.8854, 20.4361) -> (-12.094, 18.0018)
  line L161 (-12.094, 18.0018) -> (-12.5898, 17.6369)
  line L162 (-12.5898, 17.6369) -> (-14.0755, 19.6559)
  line L163 (-14.0755, 19.6559) -> (-15.3086, 18.7484)
  line L164 (-15.3086, 18.7484) -> (-15.6143, 19.1638)
  line L165 (-15.6143, 19.1638) -> (-13.8854, 20.4361)
  line L166 (-18.7606, 16.1396) -> (-18.2929, 16.618)
  line L167 (-18.2929, 16.618) -> (-17.6127, 16.3235)
  line L168 (-17.6127, 16.3235) -> (-16.7617, 17.194)
  line L169 (-16.7617, 17.194) -> (-17.0797, 17.859)
  line L170 (-17.0797, 17.859) -> (-16.6234, 18.3258)
  line L171 (-16.6234, 18.3258) -> (-15.272, 15.3479)
  line L172 (-15.272, 15.3479) -> (-15.73, 14.8794)
  line L173 (-15.73, 14.8794) -> (-18.7606, 16.1396)
  line L174 (-17.1058, 16.1042) -> (-16.0045, 15.6156)
  line L175 (-16.0045, 15.6156) -> (-16.5228, 16.7006)
  line L176 (-16.5228, 16.7006) -> (-17.1058, 16.1042)
  line L177 (-17.1902, 13.2284) -> (-17.881, 12.2232)
  spline S75 degree 2 poles (-17.881, 12.2232) (-18.0863, 11.9245) (-18.3374, 11.6658) (-18.6536, 11.5421) (-19.0225, 11.5673) (-19.1852, 11.6791) knots 0 0 0 1 2 3 4 4 4
  spline S76 degree 2 poles (-19.1852, 11.6791) (-19.3614, 11.8002) (-19.524, 12.1911) (-19.4869, 12.4051) knots 0 0 0 1 2 2 2
  spline S77 degree 2 poles (-19.4869, 12.4051) (-19.7118, 12.2214) (-20.2019, 12.1974) (-20.4201, 12.3474) knots 0 0 0 1 2 2 2
  spline S78 degree 2 poles (-20.4201, 12.3474) (-20.5924, 12.4659) (-20.8068, 12.8472) (-20.8093, 13.2577) (-20.6941, 13.4745) knots 0 0 0 1 2 3 3 3
  spline S79 degree 2 poles (-20.6941, 13.4745) (-20.6194, 13.612) (-20.2903, 14.099) knots 0 0 0 1 1 1
  line L178 (-20.2903, 14.099) -> (-19.7021, 14.9548)
  line L179 (-19.7021, 14.9548) -> (-17.1902, 13.2284)
  line L180 (-18.9537, 13.6934) -> (-19.6258, 14.1553)
  line L181 (-19.6258, 14.1553) -> (-19.9495, 13.6843)
  spline S80 degree 2 poles (-19.9495, 13.6843) (-20.139, 13.4086) (-20.1736, 13.3254) knots 0 0 0 1 1 1
  spline S81 degree 2 poles (-20.1736, 13.3254) (-20.2302, 13.1979) (-20.17, 12.9451) (-20.036, 12.853) knots 0 0 0 1 2 2 2
  spline S82 degree 2 poles (-20.036, 12.853) (-19.923, 12.7754) (-19.691, 12.7766) (-19.4748, 12.9353) (-19.2367, 13.2818) knots 0 0 0 1 2 3 3 3
  line L182 (-19.2367, 13.2818) -> (-18.9537, 13.6934)
  line L183 (-17.9563, 13.0079) -> (-18.5364, 13.4066)
  line L184 (-18.5364, 13.4066) -> (-18.7653, 13.0734)
  spline S83 degree 2 poles (-18.7653, 13.0734) (-18.9693, 12.7767) (-19.0116, 12.6987) knots 0 0 0 1 1 1
  spline S84 degree 2 poles (-19.0116, 12.6987) (-19.0839, 12.5566) (-19.0391, 12.306) (-18.9166, 12.2218) knots 0 0 0 1 2 2 2
  spline S85 degree 2 poles (-18.9166, 12.2218) (-18.7998, 12.1415) (-18.568, 12.1711) (-18.4626, 12.2875) knots 0 0 0 1 2 2 2
  spline S86 degree 2 poles (-18.4626, 12.2875) (-18.4037, 12.3569) (-18.1563, 12.7169) knots 0 0 0 1 1 1
  line L185 (-18.1563, 12.7169) -> (-17.9563, 13.0079)
  line L186 (-23.3073, 4.6904) -> (-23.3385, 4.089)
  spline S87 degree 2 poles (-23.3385, 4.089) (-23.6451, 4.0808) (-23.9745, 3.7941) (-24.0157, 3.5184) knots 0 0 0 1 2 2 2
  spline S88 degree 2 poles (-24.0157, 3.5184) (-24.0597, 3.2243) (-23.8562, 2.8885) (-23.6884, 2.8635) knots 0 0 0 1 2 2 2
  spline S89 degree 2 poles (-23.6884, 2.8635) (-23.5804, 2.8473) (-23.4122, 2.9514) (-23.3337, 3.0994) knots 0 0 0 1 2 2 2
  spline S90 degree 2 poles (-23.3337, 3.0994) (-23.2811, 3.1996) (-23.1299, 3.5669) knots 0 0 0 1 1 1
  spline S91 degree 2 poles (-23.1299, 3.5669) (-22.935, 4.0381) (-22.7285, 4.2092) knots 0 0 0 1 1 1
  spline S92 degree 2 poles (-22.7285, 4.2092) (-22.4388, 4.4502) (-22.0827, 4.3969) knots 0 0 0 1 1 1
  spline S93 degree 2 poles (-22.0827, 4.3969) (-21.8506, 4.3622) (-21.49, 4.0405) (-21.3544, 3.5176) (-21.4063, 3.1706) knots 0 0 0 1 2 3 3 3
  spline S94 degree 2 poles (-21.4063, 3.1706) (-21.4911, 2.6031) (-22.0733, 2.1029) (-22.4912, 2.1513) knots 0 0 0 1 2 2 2
  line L187 (-22.4912, 2.1513) -> (-22.4278, 2.7643)
  spline S95 degree 2 poles (-22.4278, 2.7643) (-22.1899, 2.7686) (-21.9469, 2.9954) (-21.9084, 3.2528) knots 0 0 0 1 2 2 2
  spline S96 degree 2 poles (-21.9084, 3.2528) (-21.8686, 3.5193) (-21.9543, 3.6848) knots 0 0 0 1 1 1
  spline S97 degree 2 poles (-21.9543, 3.6848) (-22.0111, 3.7919) (-22.1282, 3.8094) knots 0 0 0 1 1 1
  spline S98 degree 2 poles (-22.1282, 3.8094) (-22.2339, 3.8252) (-22.3254, 3.7473) knots 0 0 0 1 1 1
  spline S99 degree 2 poles (-22.3254, 3.7473) (-22.4395, 3.6445) (-22.7815, 2.7866) (-23.0679, 2.3949) (-23.4922, 2.2117) (-23.7794, 2.2546) knots 0 0 0 1 2 3 4 4 4
  spline S100 degree 2 poles (-23.7794, 2.2546) (-24.0368, 2.2931) (-24.4465, 2.6479) (-24.5884, 3.2071) (-24.5297, 3.5999) knots 0 0 0 1 2 3 3 3
  spline S101 degree 2 poles (-24.5297, 3.5999) (-24.4442, 4.1721) (-23.824, 4.7065) (-23.3073, 4.6904) knots 0 0 0 1 2 2 2
  line L188 (-24.7816, 0.6943) -> (-21.7349, 0.7805)
  line L189 (-21.7349, 0.7805) -> (-21.7088, -0.1415)
  line L190 (-21.7088, -0.1415) -> (-23.7716, -0.7506)
  line L191 (-23.7716, -0.7506) -> (-21.6779, -1.2329)
  line L192 (-21.6779, -1.2329) -> (-21.6518, -2.1572)
  line L193 (-21.6518, -2.1572) -> (-24.6986, -2.2433)
  line L194 (-24.6986, -2.2433) -> (-24.7147, -1.6744)
  line L195 (-24.7147, -1.6744) -> (-22.3158, -1.6065)
  line L196 (-22.3158, -1.6065) -> (-24.7317, -1.0706)
  line L197 (-24.7317, -1.0706) -> (-24.7486, -0.4761)
  line L198 (-24.7486, -0.4761) -> (-22.3666, 0.1909)
  line L199 (-22.3666, 0.1909) -> (-24.7656, 0.1254)
  line L200 (-24.7656, 0.1254) -> (-24.7816, 0.6943)
  line L201 (-23.8919, -6.7117) -> (-24.0312, -6.0573)
  line L202 (-24.0312, -6.0573) -> (-23.4092, -5.6542)
  line L203 (-23.4092, -5.6542) -> (-23.6625, -4.4635)
  line L204 (-23.6625, -4.4635) -> (-24.3923, -4.3599)
  line L205 (-24.3923, -4.3599) -> (-24.5282, -3.7213)
  line L206 (-24.5282, -3.7213) -> (-21.3004, -4.2459)
  line L207 (-21.3004, -4.2459) -> (-21.164, -4.8867)
  line L208 (-21.164, -4.8867) -> (-23.8919, -6.7117)
  line L209 (-22.9458, -5.3537) -> (-21.929, -4.7074)
  line L210 (-21.929, -4.7074) -> (-23.1194, -4.5379)
  line L211 (-23.1194, -4.5379) -> (-22.9458, -5.3537)
  line L212 (-23.4272, -8.1519) -> (-20.5983, -7.017)
  line L213 (-20.5983, -7.017) -> (-20.1156, -8.2201)
  spline S102 degree 2 poles (-20.1156, -8.2201) (-19.9331, -8.675) (-19.9219, -9.1461) (-20.2105, -9.5498) (-20.4628, -9.651) knots 0 0 0 1 2 3 3 3
  spline S103 degree 2 poles (-20.4628, -9.651) (-20.7797, -9.7781) (-21.3455, -9.5721) (-21.549, -9.2207) knots 0 0 0 1 2 2 2
  spline S104 degree 2 poles (-21.549, -9.2207) (-21.5824, -9.4494) (-21.7443, -9.7947) (-21.992, -10.1318) knots 0 0 0 1 2 2 2
  line L214 (-21.992, -10.1318) -> (-22.4056, -10.6983)
  line L215 (-22.4056, -10.6983) -> (-22.6798, -10.0148)
  line L216 (-22.6798, -10.0148) -> (-22.2284, -9.3555)
  spline S105 degree 2 poles (-22.2284, -9.3555) (-21.9876, -9.0011) (-21.8799, -8.7702) (-21.8901, -8.564) (-21.9697, -8.3657) knots 0 0 0 1 2 3 3 3
  line L217 (-21.9697, -8.3657) -> (-22.0164, -8.2492)
  line L218 (-22.0164, -8.2492) -> (-23.1979, -8.7232)
  line L219 (-23.1979, -8.7232) -> (-23.4272, -8.1519)
  line L220 (-21.5657, -8.0684) -> (-21.3962, -8.491)
  spline S106 degree 2 poles (-21.3962, -8.491) (-21.231, -8.9029) (-21.0798, -9.08) (-20.8628, -9.1281) (-20.7356, -9.0771) knots 0 0 0 1 2 3 3 3
  spline S107 degree 2 poles (-20.7356, -9.0771) (-20.5932, -9.02) (-20.4779, -8.796) (-20.5095, -8.6485) knots 0 0 0 1 2 2 2
  spline S108 degree 2 poles (-20.5095, -8.6485) (-20.5294, -8.5738) (-20.6687, -8.2267) knots 0 0 0 1 1 1
  line L221 (-20.6687, -8.2267) -> (-20.8477, -7.7804)
  line L222 (-20.8477, -7.7804) -> (-21.5657, -8.0684)
  line L223 (-21.3364, -12.6215) -> (-19.1695, -11.3111)
  line L224 (-19.1695, -11.3111) -> (-19.6371, -10.5378)
  line L225 (-19.6371, -10.5378) -> (-19.1958, -10.271)
  line L226 (-19.1958, -10.271) -> (-17.9432, -12.3424)
  line L227 (-17.9432, -12.3424) -> (-18.3845, -12.6093)
  line L228 (-18.3845, -12.6093) -> (-18.8509, -11.838)
  line L229 (-18.8509, -11.838) -> (-21.0178, -13.1483)
  line L230 (-21.0178, -13.1483) -> (-21.3364, -12.6215)
  line L231 (-19.622, -15.2002) -> (-17.2937, -13.2331)
  line L232 (-17.2937, -13.2331) -> (-15.8349, -14.9598)
  line L233 (-15.8349, -14.9598) -> (-16.2289, -15.2927)
  line L234 (-16.2289, -15.2927) -> (-17.2903, -14.0362)
  line L235 (-17.2903, -14.0362) -> (-17.8068, -14.4725)
  line L236 (-17.8068, -14.4725) -> (-16.8187, -15.642)
  line L237 (-16.8187, -15.642) -> (-17.2127, -15.9748)
  line L238 (-17.2127, -15.9748) -> (-18.2007, -14.8054)
  line L239 (-18.2007, -14.8054) -> (-18.8307, -15.3376)
  line L240 (-18.8307, -15.3376) -> (-17.7317, -16.6384)
  line L241 (-17.7317, -16.6384) -> (-18.1257, -16.9712)
  line L242 (-18.1257, -16.9712) -> (-19.622, -15.2002)
  line L243 (-15.1218, -18.2363) -> (-14.7906, -17.841)
  line L244 (-14.7906, -17.841) -> (-13.7738, -18.6929)
  line L245 (-13.7738, -18.6929) -> (-14.5526, -19.6224)
  spline S109 degree 2 poles (-14.5526, -19.6224) (-14.8213, -19.6429) (-15.566, -19.3886) (-15.8545, -19.1469) knots 0 0 0 1 2 2 2
  spline S110 degree 2 poles (-15.8545, -19.1469) (-16.2213, -18.8396) (-16.5081, -18.075) (-16.3035, -17.2736) (-16.023, -16.9388) knots 0 0 0 1 2 3 3 3
  spline S111 degree 2 poles (-16.023, -16.9388) (-15.7171, -16.5738) (-14.9349, -16.2623) (-14.5142, -16.3571) knots 0 0 0 1 2 2 2
  spline S112 degree 2 poles (-14.5142, -16.3571) (-14.1911, -16.4308) (-13.8563, -16.7113) knots 0 0 0 1 1 1
  spline S113 degree 2 poles (-13.8563, -16.7113) (-13.4218, -17.0754) (-13.2379, -17.8507) (-13.4385, -18.2312) knots 0 0 0 1 2 2 2
  line L246 (-13.4385, -18.2312) -> (-13.98, -17.9261)
  spline S114 degree 2 poles (-13.98, -17.9261) (-13.8851, -17.7116) (-13.9905, -17.2839) (-14.1935, -17.1138) knots 0 0 0 1 2 2 2
  spline S115 degree 2 poles (-14.1935, -17.1138) (-14.5034, -16.8542) (-15.1967, -16.9401) (-15.5204, -17.3265) knots 0 0 0 1 2 2 2
  spline S116 degree 2 poles (-15.5204, -17.3265) (-15.868, -17.7414) (-15.8468, -18.4685) (-15.5476, -18.7191) knots 0 0 0 1 2 2 2
  spline S117 degree 2 poles (-15.5476, -18.7191) (-15.3998, -18.843) (-15.0054, -18.9764) (-14.8299, -18.984) knots 0 0 0 1 2 2 2
  line L247 (-14.8299, -18.984) -> (-14.5823, -18.6884)
  line L248 (-14.5823, -18.6884) -> (-15.1218, -18.2363)
  line L249 (-11.5969, -20.6666) -> (-11.3424, -20.218)
  line L250 (-11.3424, -20.218) -> (-10.1886, -20.8725)
  line L251 (-10.1886, -20.8725) -> (-10.7869, -21.9273)
  spline S118 degree 2 poles (-10.7869, -21.9273) (-11.0474, -21.9959) (-11.8258, -21.8802) (-12.1532, -21.6945) knots 0 0 0 1 2 2 2
  spline S119 degree 2 poles (-12.1532, -21.6945) (-12.5695, -21.4584) (-12.9895, -20.7581) (-12.9328, -19.9329) (-12.7173, -19.553) knots 0 0 0 1 2 3 3 3
  spline S120 degree 2 poles (-12.7173, -19.553) (-12.4823, -19.1388) (-11.7691, -18.6913) (-11.3383, -18.7087) knots 0 0 0 1 2 2 2
  spline S121 degree 2 poles (-11.3383, -18.7087) (-11.0072, -18.7229) (-10.6273, -18.9384) knots 0 0 0 1 1 1
  spline S122 degree 2 poles (-10.6273, -18.9384) (-10.1342, -19.218) (-9.8135, -19.9475) (-9.9421, -20.3579) knots 0 0 0 1 2 2 2
  line L252 (-9.9421, -20.3579) -> (-10.5297, -20.1555)
  spline S123 degree 2 poles (-10.5297, -20.1555) (-10.4751, -19.9274) (-10.6559, -19.5257) (-10.8863, -19.395) knots 0 0 0 1 2 2 2
  spline S124 degree 2 poles (-10.8863, -19.395) (-11.2379, -19.1956) (-11.9043, -19.4052) (-12.153, -19.8437) knots 0 0 0 1 2 2 2
  spline S125 degree 2 poles (-12.153, -19.8437) (-12.4201, -20.3145) (-12.268, -21.0258) (-11.9285, -21.2184) knots 0 0 0 1 2 2 2
  spline S126 degree 2 poles (-11.9285, -21.2184) (-11.7608, -21.3135) (-11.3488, -21.3736) (-11.1748, -21.3494) knots 0 0 0 1 2 2 2
  line L253 (-11.1748, -21.3494) -> (-10.9846, -21.0139)
  line L254 (-10.9846, -21.0139) -> (-11.5969, -20.6666)
  line L255 (-7.5422, -23.6501) -> (-7.6945, -20.4168)
  line L256 (-7.6945, -20.4168) -> (-7.0567, -20.6115)
  line L257 (-7.0567, -20.6115) -> (-6.9754, -22.9949)
  line L258 (-6.9754, -22.9949) -> (-5.6036, -21.0551)
  line L259 (-5.6036, -21.0551) -> (-4.9792, -21.2456)
  line L260 (-4.9792, -21.2456) -> (-6.9112, -23.8428)
  line L261 (-6.9112, -23.8428) -> (-7.5422, -23.6501)
  line L262 (-3.6462, -24.0248) -> (-3.7495, -24.5586)
  line L263 (-3.7495, -24.5586) -> (-5.759, -24.1697)
  spline S127 degree 2 poles (-5.759, -24.1697) (-5.6688, -23.8748) (-5.238, -23.3974) (-4.668, -23.0439) knots 0 0 0 1 2 2 2
  spline S128 degree 2 poles (-4.668, -23.0439) (-4.2105, -22.7586) (-4.0987, -22.6453) knots 0 0 0 1 1 1
  spline S129 degree 2 poles (-4.0987, -22.6453) (-3.9456, -22.4904) (-3.9121, -22.317) knots 0 0 0 1 1 1
  spline S130 degree 2 poles (-3.9121, -22.317) (-3.875, -22.1254) (-4.0406, -21.8804) (-4.223, -21.8451) knots 0 0 0 1 2 2 2
  spline S131 degree 2 poles (-4.223, -21.8451) (-4.401, -21.8107) (-4.655, -21.9863) (-4.7195, -22.2341) knots 0 0 0 1 2 2 2
  line L264 (-4.7195, -22.2341) -> (-5.281, -22.0663)
  spline S132 degree 2 poles (-5.281, -22.0663) (-5.139, -21.6016) (-4.5208, -21.2929) (-4.1171, -21.3711) knots 0 0 0 1 2 2 2
  spline S133 degree 2 poles (-4.1171, -21.3711) (-3.6746, -21.4567) (-3.2605, -22.0314) (-3.3294, -22.3872) knots 0 0 0 1 2 2 2
  spline S134 degree 2 poles (-3.3294, -22.3872) (-3.3682, -22.5879) (-3.5825, -22.925) (-3.7787, -23.0953) knots 0 0 0 1 2 2 2
  spline S135 degree 2 poles (-3.7787, -23.0953) (-3.9093, -23.2073) (-4.5483, -23.5995) (-4.7261, -23.7354) (-4.7844, -23.8046) knots 0 0 0 1 2 3 3 3
  line L265 (-4.7844, -23.8046) -> (-3.6462, -24.0248)
  line L266 (-3.2345, -24.6144) -> (-3.1647, -24.0331)
  line L267 (-3.1647, -24.0331) -> (-2.5834, -24.1029)
  line L268 (-2.5834, -24.1029) -> (-2.6532, -24.6842)
  line L269 (-2.6532, -24.6842) -> (-3.2345, -24.6144)
  line L270 (-0.6892, -24.8203) -> (-1.274, -24.7924)
  line L271 (-1.274, -24.7924) -> (-1.1689, -22.5948)
  spline S136 degree 2 poles (-1.1689, -22.5948) (-1.5033, -22.8765) (-1.9441, -22.9997) knots 0 0 0 1 1 1
  line L272 (-1.9441, -22.9997) -> (-1.9188, -22.4706)
  spline S137 degree 2 poles (-1.9188, -22.4706) (-1.6855, -22.4073) (-1.1295, -22.0153) (-1.0164, -21.7416) knots 0 0 0 1 2 2 2
  line L273 (-1.0164, -21.7416) -> (-0.543, -21.7642)
  line L274 (-0.543, -21.7642) -> (-0.6892, -24.8203)
  point P0 (0, -0.075)
  dimension "d72" = 49.5
  constraints: 1 centre point, 1 coincident, 1 other
  measures "d72" diameter of A0
emboss "Emboss1" sketch "Sketch13" operation cut depth 0.39 direction (-1, 0, 0)
ref_plane "Work Plane2" through (0, -10.6204, -14.0095) normal (0, 0.7948428, -0.6068154) x (0, 0.6068154, 0.7948428)
equation "\"d38\" = d37"
equation "\"d41\" = 2 * Thread_Pitch"
equation "\"d50\" = 2 * Thread_Pitch"
equation "\"d68\" = d67"
body "Solid1"
body "Solid3"
